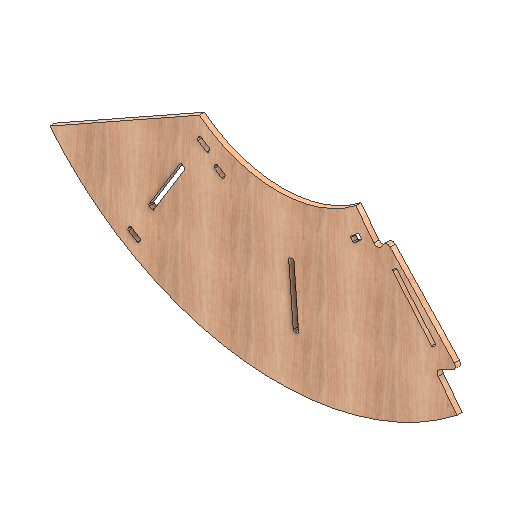
# Autodesk Inventor part: Platform B1
Saved by Autodesk Inventor 2021 (Build 250183000, 183)
## iProperties
Created: 2020-05-09
Part Number: Platform B1
Material: Wood (Birch)
Document SubType Name: Modeling
Designer: Dan Wikman
Density: 0.55 g/cm^3
Appearance: Birch - Natural Polished
Mass: 6374.12 g
Surface Area: 13840.2 cm^2
Volume: 11589.3 cm^3
Autodesk Inventor part; units mm, degrees
ref_plane "YZ Plane" through (0, 0, 0) normal (1, 0, 0) x (0, 1, 0)
ref_plane "XZ Plane" through (0, 0, 0) normal (0, 1, 0) x (-1, 0, 0)
ref_plane "XY Plane" through (0, 0, 0) normal (0, 0, 1) x (1, 0, 0)
sketch "CONTOURS" plane through (0, 0, 0) normal (0, 0, 1) x (1, 0, 0)
  line L0 (2153.8888, 619.2359) -> (2163.4719, 633.117)
  arc A0 (2185.9832, 634.7957) -> (2163.4719, 633.117) centre (2175.4045, 624.8791) ccw
  line L1 (2185.9832, 634.7957) -> (2411.1355, 394.6117)
  arc A1 (2406.7717, 371.5944) -> (2411.1355, 394.6117) centre (2400.5567, 384.695) ccw
  line L2 (2406.7717, 371.5944) -> (2360.367, 349.5799)
  arc A2 (2360.367, 349.5799) -> (2354.7432, 326.1016) centre (2367.0105, 335.5759) ccw
  line L3 (2354.7432, 326.1016) -> (2420.766, 240.6152)
  arc A3 (991.9076, 405.3519) -> (2420.766, 240.6152) centre (1790.9625, 1056.9921) ccw
  line L4 (991.9076, 405.3519) -> (1516.221, 700.5434)
  arc A4 (1516.221, 700.5434) -> (2065.5544, 700.5434) centre (1790.8877, 1057.1243) ccw
  line L5 (2065.5544, 700.5434) -> (2128.8659, 618.5677)
  arc A5 (2128.8659, 618.5677) -> (2153.8888, 619.2359) centre (2141.1332, 628.042) ccw
  constraints: 12 end point, 12 point on circle, 6 centre point
sketch "HOLES" plane through (0, 0, 0) normal (0, 0, 1) x (1, 0, 0)
  arc A0 (1449.9335, 932.975) -> (1455.5442, 933.6958) centre (1452.3785, 936.1408) ccw
  line L0 (1449.9335, 932.975) -> (1421.4416, 954.9799)
  arc A1 (1420.7208, 960.5906) -> (1421.4416, 954.9799) centre (1423.8866, 958.1456) ccw
  line L1 (1420.7208, 960.5906) -> (1427.4445, 969.2965)
  arc A2 (1433.0553, 970.0172) -> (1427.4445, 969.2965) centre (1430.6103, 966.8515) ccw
  line L2 (1433.0553, 970.0172) -> (1461.5471, 948.0124)
  arc A3 (1462.2679, 942.4017) -> (1461.5471, 948.0124) centre (1459.1022, 944.8467) ccw
  line L3 (581.1233, 599.0223) -> (574.9213, 608.1072)
  arc A4 (574.9213, 608.1072) -> (569.3624, 609.1555) centre (571.6177, 605.8519) ccw
  line L4 (569.3624, 609.1555) -> (539.6301, 588.858)
  arc A5 (539.6301, 588.858) -> (538.5818, 583.2991) centre (541.8854, 585.5544) ccw
  line L5 (538.5818, 583.2991) -> (544.7838, 574.2142)
  arc A6 (544.7838, 574.2142) -> (550.3427, 573.1659) centre (548.0874, 576.4695) ccw
  line L6 (550.3427, 573.1659) -> (580.075, 593.4634)
  arc A7 (580.075, 593.4634) -> (581.1233, 599.0223) centre (577.8197, 596.767) ccw
  line L7 (1171.3736, 565.7512) -> (1178.0973, 574.4571)
  arc A8 (1178.0973, 574.4571) -> (1177.3765, 580.0678) centre (1174.9316, 576.9021) ccw
  line L8 (1177.3765, 580.0678) -> (1148.8847, 602.0727)
  arc A9 (1148.8847, 602.0727) -> (1143.2739, 601.3519) centre (1146.4397, 598.9069) ccw
  line L9 (1143.2739, 601.3519) -> (1136.5502, 592.646)
  arc A10 (1136.5502, 592.646) -> (1137.271, 587.0353) centre (1139.716, 590.201) ccw
  line L10 (1137.271, 587.0353) -> (1165.7629, 565.0304)
  arc A11 (1165.7629, 565.0304) -> (1171.3736, 565.7512) centre (1168.2079, 568.1962) ccw
  line L11 (312.7987, 992.0706) -> (319.0007, 982.9857)
  arc A12 (317.9524, 977.4269) -> (319.0007, 982.9857) centre (315.6972, 980.7305) ccw
  line L12 (317.9524, 977.4269) -> (288.2201, 957.1293)
  arc A13 (282.6613, 958.1776) -> (288.2201, 957.1293) centre (285.9648, 960.4329) ccw
  line L13 (282.6613, 958.1776) -> (276.4592, 967.2625)
  arc A14 (277.5075, 972.8214) -> (276.4592, 967.2625) centre (279.7628, 969.5178) ccw
  line L14 (277.5075, 972.8214) -> (307.2399, 993.1189)
  arc A15 (312.7987, 992.0706) -> (307.2399, 993.1189) centre (309.4951, 989.8153) ccw
  arc A16 (877.4586, 807.9096) -> (881.5741, 811.7907) centre (877.5758, 811.9079) ccw
  line L15 (881.5741, 811.7907) -> (887.6999, 1020.7009)
  arc A17 (887.6999, 1020.7009) -> (883.8189, 1024.8164) centre (883.7016, 1020.8181) ccw
  line L16 (883.8189, 1024.8164) -> (872.8236, 1025.1388)
  arc A18 (872.8236, 1025.1388) -> (868.7081, 1021.2578) centre (872.7064, 1021.1405) ccw
  line L17 (868.7081, 1021.2578) -> (862.5822, 812.3476)
  arc A19 (862.5822, 812.3476) -> (866.4633, 808.232) centre (866.5805, 812.2303) ccw
  line L18 (866.4633, 808.232) -> (877.4586, 807.9096)
  arc A20 (370.076, 874.2818) -> (369.0277, 868.7229) centre (372.3312, 870.9782) ccw
  line L19 (369.0277, 868.7229) -> (486.8661, 696.1104)
  arc A21 (486.8661, 696.1104) -> (492.425, 695.062) centre (490.1697, 698.3656) ccw
  line L20 (492.425, 695.062) -> (501.5098, 701.2641)
  arc A22 (501.5098, 701.2641) -> (502.5581, 706.8229) centre (499.2546, 704.5677) ccw
  line L21 (502.5581, 706.8229) -> (384.7197, 879.4355)
  arc A23 (384.7197, 879.4355) -> (379.1608, 880.4838) centre (381.4161, 877.1802) ccw
  line L22 (379.1608, 880.4838) -> (370.076, 874.2818)
  line L23 (1833.6661, 426.4523) -> (1844.634, 427.2924)
  arc A24 (1833.6661, 426.4523) -> (1829.9832, 422.1586) centre (1833.9716, 422.464) ccw
  line L24 (1845.9439, 213.7689) -> (1829.9832, 422.1586)
  arc A25 (1101.2975, 659.9143) -> (1095.6868, 659.1936) centre (1098.8525, 656.7486) ccw
  arc A26 (1845.9439, 213.7689) -> (1850.2377, 210.086) centre (1849.9322, 214.0744) ccw
  arc A27 (2077.5111, 618.774) -> (2071.8727, 619.2297) centre (2074.4641, 616.1826) ccw
  line L25 (620.0838, 641.0058) -> (644.8608, 657.9204)
  arc A28 (644.8608, 657.9204) -> (645.9091, 663.4793) centre (642.6055, 661.224) ccw
  line L26 (645.9091, 663.4793) -> (639.707, 672.5642)
  arc A29 (639.707, 672.5642) -> (634.1482, 673.6125) centre (636.4035, 670.3089) ccw
  line L27 (634.1482, 673.6125) -> (609.3712, 656.6979)
  arc A30 (609.3712, 656.6979) -> (608.3229, 651.139) centre (611.6265, 653.3943) ccw
  line L28 (608.3229, 651.139) -> (614.525, 642.0541)
  arc A31 (614.525, 642.0541) -> (620.0838, 641.0058) centre (617.8286, 644.3094) ccw
  line L29 (1089.6839, 644.877) -> (1113.4271, 626.5396)
  arc A32 (1113.4271, 626.5396) -> (1119.0379, 627.2604) centre (1115.8721, 629.7054) ccw
  line L30 (1119.0379, 627.2604) -> (1125.7616, 635.9662)
  arc A33 (1125.7616, 635.9662) -> (1125.0408, 641.577) centre (1122.5958, 638.4112) ccw
  line L31 (1125.0408, 641.577) -> (1101.2975, 659.9143)
  arc A34 (1553.2327, 613.0929) -> (1551.9237, 618.5962) centre (1549.8265, 615.19) ccw
  line L32 (1095.6868, 659.1936) -> (1088.9631, 650.4877)
  arc A35 (1088.9631, 650.4877) -> (1089.6839, 644.877) centre (1092.1288, 648.0427) ccw
  line L33 (1266.2545, 230.909) -> (1272.0216, 240.2759)
  arc A36 (1277.5249, 241.5849) -> (1272.0216, 240.2759) centre (1275.4278, 238.1788) ccw
  line L34 (1277.5249, 241.5849) -> (1308.1804, 222.7106)
  arc A37 (1309.4894, 217.2073) -> (1308.1804, 222.7106) centre (1306.0833, 219.3045) ccw
  line L35 (1309.4894, 217.2073) -> (1303.7223, 207.8403)
  arc A38 (1298.219, 206.5313) -> (1303.7223, 207.8403) centre (1300.3161, 209.9375) ccw
  line L36 (1298.219, 206.5313) -> (1267.5635, 225.4056)
  arc A39 (1266.2545, 230.909) -> (1267.5635, 225.4056) centre (1269.6606, 228.8118) ccw
  line L37 (1515.7649, 636.1615) -> (1509.9977, 626.7945)
  arc A40 (1509.9977, 626.7945) -> (1511.3067, 621.2912) centre (1513.4039, 624.6974) ccw
  line L38 (1511.3067, 621.2912) -> (1541.9622, 602.4169)
  arc A41 (1541.9622, 602.4169) -> (1547.4655, 603.7259) centre (1544.0594, 605.8231) ccw
  line L39 (1547.4655, 603.7259) -> (1553.2327, 613.0929)
  line L40 (1551.9237, 618.5962) -> (1521.2682, 637.4705)
  arc A42 (1521.2682, 637.4705) -> (1515.7649, 636.1615) centre (1519.171, 634.0643) ccw
  line L41 (2048.564, 594.1557) -> (2055.6903, 585.7762)
  arc A43 (2055.6903, 585.7762) -> (2061.3288, 585.3206) centre (2058.7374, 588.3676) ccw
  line L42 (2061.3288, 585.3206) -> (2084.1818, 604.7561)
  arc A44 (2084.1818, 604.7561) -> (2084.6375, 610.3946) centre (2081.5904, 607.8032) ccw
  line L43 (2084.6375, 610.3946) -> (2077.5111, 618.774)
  line L44 (2071.8727, 619.2297) -> (2049.0196, 599.7942)
  arc A45 (2049.0196, 599.7942) -> (2048.564, 594.1557) centre (2051.611, 596.7471) ccw
  arc A46 (2196.184, 571.948) -> (2195.7283, 566.3095) centre (2198.7754, 568.9009) ccw
  line L45 (2195.7283, 566.3095) -> (2331.1291, 407.1002)
  arc A47 (2331.1291, 407.1002) -> (2336.7676, 406.6445) centre (2334.1762, 409.6916) ccw
  line L46 (2336.7676, 406.6445) -> (2345.147, 413.7708)
  arc A48 (2345.147, 413.7708) -> (2345.6027, 419.4093) centre (2342.5556, 416.8179) ccw
  line L47 (2345.6027, 419.4093) -> (2210.2019, 578.6187)
  arc A49 (2210.2019, 578.6187) -> (2204.5634, 579.0743) centre (2207.1548, 576.0273) ccw
  line L48 (2204.5634, 579.0743) -> (2196.184, 571.948)
  arc A50 (1339.7556, 342.3599) -> (1341.0646, 336.8566) centre (1343.1618, 340.2628) ccw
  line L49 (1339.7556, 342.3599) -> (1449.3315, 520.3322)
  arc A51 (1454.8349, 521.6412) -> (1449.3315, 520.3322) centre (1452.7377, 518.235) ccw
  line L50 (1454.8349, 521.6412) -> (1464.2018, 515.874)
  arc A52 (1465.5108, 510.3707) -> (1464.2018, 515.874) centre (1462.1047, 512.4678) ccw
  line L51 (1465.5108, 510.3707) -> (1355.9349, 332.3985)
  arc A53 (1350.4316, 331.0895) -> (1355.9349, 332.3985) centre (1352.5287, 334.4956) ccw
  line L52 (1350.4316, 331.0895) -> (1341.0646, 336.8566)
  line L53 (1462.2679, 942.4017) -> (1455.5442, 933.6958)
  arc A54 (1606.7292, 560.351) -> (1605.4201, 565.8543) centre (1603.323, 562.4481) ccw
  line L54 (1579.8739, 581.5829) -> (1605.4201, 565.8543)
  arc A55 (1579.8739, 581.5829) -> (1574.3706, 580.2739) centre (1577.7767, 578.1767) ccw
  line L55 (1568.6034, 570.9069) -> (1574.3706, 580.2739)
  arc A56 (1568.6034, 570.9069) -> (1569.9124, 565.4036) centre (1572.0096, 568.8098) ccw
  line L56 (1595.4587, 549.675) -> (1569.9124, 565.4036)
  arc A57 (1595.4587, 549.675) -> (1600.962, 550.984) centre (1597.5558, 553.0812) ccw
  line L57 (1606.7292, 560.351) -> (1600.962, 550.984)
  line L58 (1861.2056, 210.9261) -> (1850.2377, 210.086)
  arc A58 (1861.2056, 210.9261) -> (1864.8884, 215.2199) centre (1860.9001, 214.9144) ccw
  line L59 (1848.9278, 423.6095) -> (1864.8884, 215.2199)
  arc A59 (1848.9278, 423.6095) -> (1844.634, 427.2924) centre (1844.9394, 423.3041) ccw
  dimension "d13" = 122.5342
  dimension "d15" = 116.3458
  dimension "d17" = 116.3234
  dimension "d19" = 19
  dimension "d21" = 122.5114
  dimension "d23" = 30
  dimension "d25" = 36
  dimension "d27" = 36
  dimension "d29" = 29
  constraints: 120 end point, 120 point on circle, 60 centre point
  measures "d13" distance of L37.end L49.end
  measures "d15" distance of L38.end L50.end
  measures "d17" distance of L52.start L34.end
  measures "d19" distance between parallel lines of L34 L36
  measures "d21" distance of L49.start L33.end
  measures "d23" distance of L54.start L54.end
  measures "d25" distance of L34.start L34.end
  measures "d27" angle of L24 L51
sketch "LETTERS" plane through (0, 0, 0) normal (0, 0, 1) x (1, 0, 0)
  line L0 (1512.6274, 378.3219) -> (1504.8915, 360.2317)
  line L1 (1504.8915, 360.2317) -> (1513.0744, 356.7244)
  arc A0 (1517.2734, 366.5323) -> (1520.8186, 374.8004) centre (1519.042, 370.668) ccw
  line L2 (1517.2734, 366.5323) -> (1509.1534, 370.0046)
  arc A1 (1513.0744, 356.7244) -> (1517.2734, 366.5323) centre (1515.1759, 361.6275) ccw
  line L3 (1520.8186, 374.8004) -> (1512.6274, 378.3219)
  constraints: 8 end point, 4 point on circle, 4 tangent, 2 centre point
extrude "Extrusion2" add sketch "CONTOURS" along normal blind 18
extrude "Extrusion3" cut sketch "HOLES" along normal blind 18 contours L23 A59 L59 A58 L58 A26 L24 A24 | L43 A44 L42 A43 L41 A45 L44 A27 | L39 A41 L38 A40 L37 A42 L40 A34 | L33 A36 L34 A37 L35 A38 L36 A39 | L48 A49 L47 A48 L46 A47 L45 A46 | L49 A51 L50 A52 L51 A53 L52 A50 | L57 A57 L56 A56 L55 A55 L54 A54
body "Solid2"
